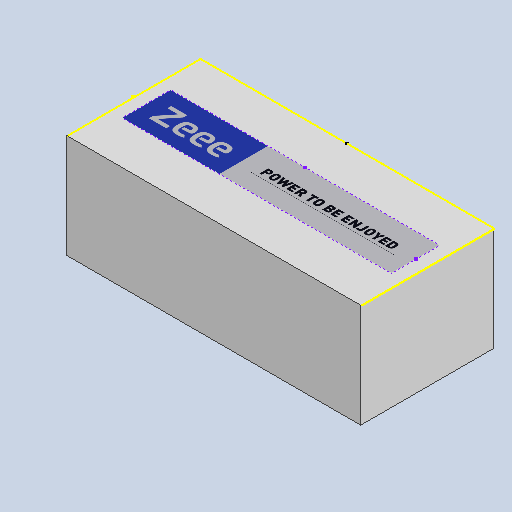
# Autodesk Inventor part: battery
Saved by Autodesk Inventor 2024 (Build 280153000, 153)
## iProperties
Created: 2023-10-20
Part Number: battery
Material: Generic
Document SubType Name: Modeling
Designer: kdcao
Density: 1 g/cm^3
Appearance: Default
Author: kdcao
Autodesk Inventor part; units mm, degrees
ref_plane "YZ Plane" through (0, 0, 0) normal (1, 0, 0) x (0, 1, 0)
ref_plane "XZ Plane" through (0, 0, 0) normal (0, 1, 0) x (-1, 0, 0)
ref_plane "XY Plane" through (0, 0, 0) normal (0, 0, 1) x (1, 0, 0)
sketch "Sketch1" plane through (0, 0, 0) normal (1, 0, 0) x (0, 1, 0)
  line L0 (-13.25, 17) -> (13.25, 17)
  line L1 (13.25, 17) -> (13.25, -17)
  line L2 (13.25, -17) -> (-13.25, -17)
  line L3 (-13.25, -17) -> (-13.25, 17)
  line L4 (-13.25, 17) -> (13.25, -17) construction
  line L5 (13.25, 17) -> (-13.25, -17) construction
  point P0 (0, 0)
  dimension "d0" = 34
  dimension "d1" = 26.5
  constraints: 12 end point, 2 midpoint, 2 parallel, 1 horizontal, 1 perpendicular
  measures "d0" distance of L0.end L1.end
  measures "d1" distance of L0.start L0.end
extrude "Extrusion1" add sketch "Sketch1" along normal blind 75
sketch "Sketch2" plane through (0, 13.25, 17) normal (0, 1, 0) x (1, 0, 0)
  line L0 (3.1206, 23.3836) -> (71.8794, 23.3836) construction
  line L1 (71.8794, 23.3836) -> (71.8794, 10.9341) construction
  line L2 (71.8794, 10.9341) -> (3.1206, 10.9341) construction
  line L3 (3.1206, 10.9341) -> (3.1206, 23.3836) construction
  line L4 (0, 34) -> (75, 34) projected
  line L5 (0, 34) -> (0, 0) projected
  line L6 (75, 34) -> (75, 0) projected
  point P0 (0, 17)
  point P1 (37.5, 34)
  point P2 (37.5, 23.3836)
  point P3 (71.8794, 17.1588)
  constraints: 3 midpoint, 2 other
body "Solid1"
